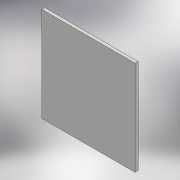
# Autodesk Inventor part: bottom
Saved by Autodesk Inventor 2017 (Build 210142000, 142)
## iProperties
Created: 2017-03-04
Part Number: bottom
Material: Generic
Document SubType Name: Modeling
Designer: dpgai
Density: 1 g/cm^3
Appearance: Default
Author: dpgai
Autodesk Inventor part; units mm, degrees
ref_plane "YZ Plane" through (0, 0, 0) normal (1, 0, 0) x (0, 1, 0)
ref_plane "XZ Plane" through (0, 0, 0) normal (0, 1, 0) x (-1, 0, 0)
ref_plane "XY Plane" through (0, 0, 0) normal (0, 0, 1) x (1, 0, 0)
sketch "Sketch1" plane through (0, 0, 0) normal (0, 1, 0) x (-1, 0, 0)
  line L0 (0, 0) -> (98.481, 0)
  line L1 (98.481, 0) -> (98.481, -100)
  line L2 (98.481, -100) -> (0, -100)
  line L3 (0, -100) -> (0, 0)
  dimension "d0" = 98.481
  dimension "d1" = 100
  constraints: 8 end point, 2 parallel, 1 horizontal, 1 perpendicular
  measures "d0" distance of L1.end L2.end
  measures "d1" distance of L0.end L1.end
extrude "Extrusion1" add sketch "Sketch1" along normal blind 3.175
body "Solid1"
